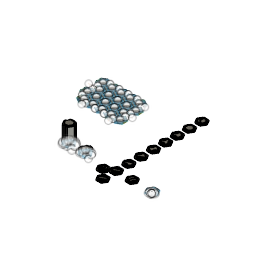
OpenHexTiles (Autodesk Fusion 360 design; units mm, degrees)
part number: 2025-10-27-16-40-17-945
part number: 2025-10-29-18-29-54-015
part number: 2025-10-29-18-44-09-003
part number: 2025-11-06-19-48-26-716
part number: 2025-11-07-19-21-59-291
part number: 2025-11-23-17-37-19-176
part number: 2025-11-23-17-48-45-361
part number: 2025-11-23-18-24-08-497
part number: 2025-11-24-19-12-39-372
part number: 2025-11-24-19-25-12-724
part number: 2025-11-24-19-31-14-734
part number: 2025-11-24-19-34-23-874
part number: 2025-11-24-19-39-51-757
part number: 2025-11-24-19-43-10-627
part number: 2025-11-24-19-46-33-060
part number: 2025-11-24-19-51-15-923
Autodesk Fusion 360 part; units mm, degrees
(part 1 of 3)
sketch "Main Hex Tile" plane through (0, 0, 0) normal (0, 0, 1) x (1, 0, 0) in component "Basic Hext Tile"
  line L0 (19.8352, 0.961) -> (10.3609, 17.371)
  line L1 (10.3609, 17.371) -> (-8.5878, 17.371)
  line L2 (-8.5878, 17.371) -> (-18.0621, 0.961)
  line L3 (-18.0621, 0.961) -> (-8.5878, -15.449)
  line L4 (-8.5878, -15.449) -> (10.3609, -15.449)
  line L5 (10.3609, -15.449) -> (19.8352, 0.961)
  line L6 (14.743, 0.961) -> (7.8148, 12.961)
  line L7 (7.8148, 12.961) -> (-6.0416, 12.961)
  line L8 (-6.0416, 12.961) -> (-12.9698, 0.961)
  line L9 (-12.9698, 0.961) -> (-6.0416, -11.039)
  line L10 (-6.0416, -11.039) -> (7.8148, -11.039)
  line L11 (7.8148, -11.039) -> (14.743, 0.961)
  line L12 (15.098, -7.244) -> (23.6888, -12.2039) construction
  line L13 (16.7724, -4.344) -> (13.4237, -10.144)
  line L14 (13.4237, -10.144) -> (14.9248, -12.744)
  line L15 (14.9248, -12.744) -> (19.7746, -4.344)
  line L16 (19.7746, -4.344) -> (16.7724, -4.344)
  line L17 (0.8866, -15.449) -> (0.8866, -15.2915) construction
  line L18 (0.8866, -15.2915) -> (0.8866, -9) construction
  line L19 (4.3866, -15.449) -> (6.1186, -12.449)
  line L20 (6.1186, -12.449) -> (-4.3455, -12.449)
  line L21 (-4.3455, -12.449) -> (-2.6134, -15.449)
  line L22 (5.7363, 19.971) -> (-3.9632, 19.971)
  line L23 (-3.9632, 19.971) -> (-2.4621, 17.371)
  line L24 (4.2352, 17.371) -> (5.7363, 19.971)
  line L25 (13.348, 12.1971) -> (9.8839, 12.1971)
  line L26 (9.8839, 12.1971) -> (15.116, 3.1349)
  line L27 (15.116, 3.1349) -> (16.848, 6.1349)
  line L28 (-18.0015, -4.344) -> (-13.1517, -12.744)
  line L29 (-13.1517, -12.744) -> (-11.6506, -10.144)
  line L30 (-14.9992, -4.344) -> (-18.0015, -4.344)
  line L31 (-15.0749, 6.1349) -> (-13.3429, 3.1349)
  line L32 (-13.3429, 3.1349) -> (-8.1108, 12.1971)
  line L33 (-8.1108, 12.1971) -> (-11.5749, 12.1971)
  line L34 (7.8725, 13.061) -> (-6.0994, 13.061)
  line L35 (-6.0994, 13.061) -> (-13.0853, 0.961)
  line L36 (-13.0853, 0.961) -> (-6.0994, -11.139)
  line L37 (-6.0994, -11.139) -> (7.8725, -11.139)
  line L38 (7.8725, -11.139) -> (14.8584, 0.961)
  line L39 (14.8584, 0.961) -> (7.8725, 13.061)
  point P0 (0.8866, 0.961)
  dimension "d4" = 32.82
  dimension "d29" = 5.8
  dimension "d31" = 2.6
  dimension "d32" = 60
  dimension "d34" = 7
  dimension "d35" = 60
  dimension "d37" = 360
  dimension "d44" = 3
  dimension "d59" = 0.1
  constraint horizontal L1
  constraint midpoint L5 L12.start
  constraint perpendicular L5 L12
  constraint perpendicular L12 L13
  constraint perpendicular L12 L15
  constraint midpoint L5 L13
  constraint symmetric L12 L14 L16
  constraint midpoint L4 L17.start
  constraint perpendicular L10 L17
  constraint perpendicular L10 L18
  constraint coincident L4 L21.end
  constraint coincident L4 L19.start
  constraint symmetric L18 L19 L21
  measures "d4" distance of L1 L4
  measures "d29" vertical distance of L13.start L13.end
  measures "d31" distance of L5 L15.end
  measures "d32" angle of L15 L16
  measures "d34" distance of L21.end L19.start
  measures "d35" angle of L20 L21
  measures "d44" distance of L4 L20
extrude "Dar Volumen" add sketch "Main Hex Tile" along normal blind 15 contours L0 L1 L2 L3 L4 L5 L13 L19 L20 L21 L25 L26 L27 L31 L32 L33 | L5 L13 L14 L15 L16 | L1 L22 L23 L24 | L3 L28 L29 L30 | L6 L7 L8 L9 L10 L11 | L34 L35 L36 L37 L38 L39 makes body 1 in component "Basic Hext Tile"
extrude "Recorte Labio Superior" cut sketch "Main Hex Tile" against normal blind 2 from surface at 15 contours L0 L1 L2 L3 L4 L5 L13 L19 L20 L21 L25 L26 L27 L31 L32 L33 | L5 L13 L14 L15 L16 | L1 L22 L23 L24 | L3 L28 L29 L30 | L34 L35 L36 L37 L38 L39 bodies 1 in component "Basic Hext Tile"
extrude "Machos" cut sketch "Main Hex Tile" along normal blind 6 contours L5 L13 L14 L15 L16 | L1 L22 L23 L24 | L3 L28 L29 L30 bodies 1 in component "Basic Hext Tile"
extrude "Extrude8" cut sketch "Main Hex Tile" along normal blind 11 contours L34 L35 L36 L37 L38 L39 bodies 1 in component "Basic Hext Tile"
extrude "Extrude9" cut sketch "Main Hex Tile" along normal blind 11 contours L6 L7 L8 L9 L10 L11 bodies 1 in component "Basic Hext Tile"
sketch "Basic Cap (Text)" plane through (0, 0, 0) normal (0, 0, 1) x (1, 0, 0) in component "Basic Cap (Text)"
  line L0 (30.6963, -0.205) -> (40.1706, -16.615)
  line L1 (40.1706, -16.615) -> (59.1192, -16.615)
  line L2 (59.1192, -16.615) -> (68.5936, -0.205)
  line L3 (68.5936, -0.205) -> (59.1192, 16.205)
  line L4 (59.1192, 16.205) -> (40.1706, 16.205)
  line L5 (40.1706, 16.205) -> (30.6963, -0.205)
  line L6 (42.7167, 11.795) -> (35.7885, -0.205)
  line L7 (35.7885, -0.205) -> (42.7167, -12.205)
  line L8 (42.7167, -12.205) -> (56.5731, -12.205)
  line L9 (56.5731, -12.205) -> (63.5013, -0.205)
  line L10 (63.5013, -0.205) -> (56.5731, 11.795)
  line L11 (56.5731, 11.795) -> (42.7167, 11.795)
  line L12 (42.659, 11.895) -> (35.6731, -0.205)
  line L13 (35.6731, -0.205) -> (42.659, -12.305)
  line L14 (42.659, -12.305) -> (56.6309, -12.305)
  line L15 (56.6309, -12.305) -> (63.6168, -0.205)
  line L16 (63.6168, -0.205) -> (56.6309, 11.895)
  line L17 (56.6309, 11.895) -> (42.659, 11.895)
  line L18 (36.7542, -3.3815) -> (62.5357, -3.3815) construction
  line L19 (62.5357, -3.3815) -> (62.5357, 2.9715) construction
  line L20 (62.5357, 2.9715) -> (36.7542, 2.9715) construction
  line L21 (36.7542, 2.9715) -> (36.7542, -3.3815) construction
  line L22 (49.6449, 11.795) -> (49.6449, -12.205) construction
  line L23 (60.0372, 5.795) -> (39.2526, -6.205) construction
  line L24 (39.166, 5.845) -> (60.1238, -6.255) construction
  line L25 (36.8278, -0.205) -> (43.2363, -11.305)
  line L26 (43.2363, -11.305) -> (56.0535, -11.305)
  line L27 (56.0535, -11.305) -> (62.4621, -0.205)
  line L28 (62.4621, -0.205) -> (56.0535, 10.895)
  line L29 (56.0535, 10.895) -> (43.2363, 10.895)
  line L30 (43.2363, 10.895) -> (36.8278, -0.205)
  point P0 (49.6449, -0.205)
  dimension "d65_1" = 32.82
  dimension "d67_1" = 0.1
  dimension "d88" = 4
  dimension "d89" = 0
  text T0 "+3\nWATER3\nPSR+1" font "Arial" height 4 bold align centre middle in box 25.7815 x 6.353 at (36.7542, -3.3815) x (1, 0) y (0, 1) spacing 1 kerned
  constraint horizontal L4
  constraint midpoint L11 L22.start
  constraint midpoint L8 L22.end
  constraint midpoint L10 L23.start
  constraint midpoint L7 L23.end
  constraint midpoint L12 L24.start
  constraint midpoint L15 L24.end
  constraint coincident P0
  constraint horizontal L20
  measures "d65_1" distance of L1 L4
extrude "Main Cap Body" add sketch "Basic Cap (Text)" sketch "Basic Cap (Text)" along normal blind 4.8 separate body contours L0 L1 L2 L3 L4 L5 | L6 L7 L8 L9 L10 L11 | L12 L13 L14 L15 L16 L17 | L25 L26 L27 L28 L29 L30 of sketch 2 text T0 makes body 2 in component "Basic Cap (Text)"
extrude "Outside lip cut" cut sketch "Basic Cap (Text)" against normal blind 1.8 from surface at 4.8 contours L0 L1 L2 L3 L4 L5 | L12 L13 L14 L15 L16 L17 bodies 2 in component "Basic Cap (Text)"
extrude "Hole for text" cut sketch "Basic Cap (Text)" against normal blind 1.2 from surface at 4.8 contours L25 L26 L27 L28 L29 L30 bodies 2 in component "Basic Cap (Text)"
extrude "Internal Hole" cut sketch "Basic Cap (Text)" along normal blind 2 contours L6 L7 L8 L9 L10 L11 | L12 L13 L14 L15 L16 L17 | L25 L26 L27 L28 L29 L30 bodies 2 in component "Basic Cap (Text)"
extrude "Text" add sketch "Basic Cap (Text)" along normal blind 1.2 from surface at 3.6 text T0 bodies 2 in component "Basic Cap (Text)"
sketch "Slab" plane through (0, 0, 0) normal (0, 0, 1) x (1, 0, 0) in component "Slab"
  line L0 (-173.2109, 149.9603) -> (-156.8009, 159.4346)
  line L1 (-189.6209, 178.3833) -> (-189.6209, 159.4346)
  line L2 (-189.6209, 159.4346) -> (-173.2109, 149.9603)
  line L3 (-185.2109, 175.8372) -> (-185.2109, 161.9807)
  line L4 (-185.2109, 161.9807) -> (-173.2109, 155.0525)
  line L5 (-173.2109, 155.0525) -> (-161.2109, 161.9807)
  line L6 (-161.2109, 161.9807) -> (-161.2109, 175.8372)
  line L7 (-161.2109, 175.8372) -> (-173.2109, 182.7654)
  line L8 (-173.2109, 182.7654) -> (-185.2109, 175.8372)
  line L9 (-152.3909, 175.8372) -> (-152.3909, 161.9807)
  line L10 (-140.3909, 182.7654) -> (-152.3909, 175.8372)
  line L11 (-128.3909, 175.8372) -> (-140.3909, 182.7654)
  line L12 (-152.3909, 161.9807) -> (-140.3909, 155.0525)
  line L13 (-140.3909, 155.0525) -> (-128.3909, 161.9807)
  line L14 (-128.3909, 161.9807) -> (-128.3909, 175.8372)
  line L15 (-156.8009, 159.4346) -> (-140.3909, 149.9603)
  line L16 (-140.3909, 149.9603) -> (-123.9809, 159.4346)
  line L17 (-119.5709, 175.8372) -> (-119.5709, 161.9807)
  line L18 (-107.5709, 182.7654) -> (-119.5709, 175.8372)
  line L19 (-95.5709, 175.8372) -> (-107.5709, 182.7654)
  line L20 (-119.5709, 161.9807) -> (-107.5709, 155.0525)
  line L21 (-107.5709, 155.0525) -> (-95.5709, 161.9807)
  line L22 (-95.5709, 161.9807) -> (-95.5709, 175.8372)
  line L23 (-123.9809, 159.4346) -> (-107.5709, 149.9603)
  line L24 (-107.5709, 149.9603) -> (-91.1609, 159.4346)
  line L25 (-86.7509, 175.8372) -> (-86.7509, 161.9807)
  line L26 (-74.7509, 182.7654) -> (-86.7509, 175.8372)
  line L27 (-62.7509, 175.8372) -> (-74.7509, 182.7654)
  line L28 (-86.7509, 161.9807) -> (-74.7509, 155.0525)
  line L29 (-74.7509, 155.0525) -> (-62.7509, 161.9807)
  line L30 (-62.7509, 161.9807) -> (-62.7509, 175.8372)
  line L31 (-91.1609, 159.4346) -> (-74.7509, 149.9603)
  line L32 (-74.7509, 149.9603) -> (-58.3409, 159.4346)
  line L33 (-53.9309, 175.8372) -> (-53.9309, 161.9807)
  line L34 (-41.9309, 182.7654) -> (-53.9309, 175.8372)
  line L35 (-29.9309, 175.8372) -> (-41.9309, 182.7654)
  line L36 (-25.5209, 178.3833) -> (-41.9309, 187.8576)
  line L37 (-53.9309, 161.9807) -> (-41.9309, 155.0525)
  line L38 (-41.9309, 155.0525) -> (-29.9309, 161.9807)
  line L39 (-29.9309, 161.9807) -> (-29.9309, 175.8372)
  line L40 (-58.3409, 159.4346) -> (-41.9309, 149.9603)
  line L41 (-25.5209, 159.4346) -> (-25.5209, 178.3833)
  line L42 (-41.9309, 149.9603) -> (-25.5209, 159.4346)
  line L43 (-189.6209, 216.2805) -> (-206.0309, 206.8062)
  line L44 (-206.0309, 206.8062) -> (-206.0309, 187.8576)
  line L45 (-206.0309, 187.8576) -> (-189.6209, 178.3833)
  line L46 (-201.6209, 204.2601) -> (-201.6209, 190.4037)
  line L47 (-201.6209, 190.4037) -> (-189.6209, 183.4755)
  line L48 (-189.6209, 183.4755) -> (-177.6209, 190.4037)
  line L49 (-177.6209, 190.4037) -> (-177.6209, 204.2601)
  line L50 (-177.6209, 204.2601) -> (-189.6209, 211.1883)
  line L51 (-189.6209, 211.1883) -> (-201.6209, 204.2601)
  line L52 (-144.8009, 204.2601) -> (-156.8009, 211.1883)
  line L53 (-168.8009, 204.2601) -> (-168.8009, 190.4037)
  line L54 (-144.8009, 190.4037) -> (-144.8009, 204.2601)
  line L55 (-156.8009, 183.4755) -> (-144.8009, 190.4037)
  line L56 (-168.8009, 190.4037) -> (-156.8009, 183.4755)
  line L57 (-156.8009, 211.1883) -> (-168.8009, 204.2601)
  line L58 (-111.9809, 204.2601) -> (-123.9809, 211.1883)
  line L59 (-135.9809, 204.2601) -> (-135.9809, 190.4037)
  line L60 (-111.9809, 190.4037) -> (-111.9809, 204.2601)
  line L61 (-123.9809, 183.4755) -> (-111.9809, 190.4037)
  line L62 (-135.9809, 190.4037) -> (-123.9809, 183.4755)
  line L63 (-123.9809, 211.1883) -> (-135.9809, 204.2601)
  line L64 (-79.1609, 204.2601) -> (-91.1609, 211.1883)
  line L65 (-103.1609, 204.2601) -> (-103.1609, 190.4037)
  line L66 (-79.1609, 190.4037) -> (-79.1609, 204.2601)
  line L67 (-91.1609, 183.4755) -> (-79.1609, 190.4037)
  line L68 (-103.1609, 190.4037) -> (-91.1609, 183.4755)
  line L69 (-91.1609, 211.1883) -> (-103.1609, 204.2601)
  line L70 (-46.3409, 204.2601) -> (-58.3409, 211.1883)
  line L71 (-70.3409, 204.2601) -> (-70.3409, 190.4037)
  line L72 (-46.3409, 190.4037) -> (-46.3409, 204.2601)
  line L73 (-41.9309, 187.8576) -> (-41.9309, 206.8062)
  line L74 (-58.3409, 183.4755) -> (-46.3409, 190.4037)
  line L75 (-70.3409, 190.4037) -> (-58.3409, 183.4755)
  line L76 (-58.3409, 211.1883) -> (-70.3409, 204.2601)
  line L77 (-128.3909, 218.8266) -> (-128.3909, 232.683)
  line L78 (-201.6209, 261.106) -> (-201.6209, 247.2496)
  line L79 (-140.3909, 211.8984) -> (-128.3909, 218.8266)
  line L80 (-168.8009, 261.106) -> (-168.8009, 247.2496)
  line L81 (-86.7509, 218.8266) -> (-74.7509, 211.8984)
  line L82 (-152.3909, 218.8266) -> (-140.3909, 211.8984)
  line L83 (-95.5709, 218.8266) -> (-95.5709, 232.683)
  line L84 (-189.6209, 235.2292) -> (-189.6209, 216.2805)
  line L85 (-206.0309, 263.6521) -> (-206.0309, 244.7035)
  line L86 (-177.6209, 247.2496) -> (-177.6209, 261.106)
  line L87 (-189.6209, 268.0342) -> (-201.6209, 261.106)
  line L88 (-156.8009, 273.1264) -> (-173.2109, 263.6521)
  line L89 (-201.6209, 247.2496) -> (-189.6209, 240.3214)
  line L90 (-144.8009, 247.2496) -> (-144.8009, 261.106)
  line L91 (-173.2109, 263.6521) -> (-189.6209, 273.1264)
  line L92 (-74.7509, 211.8984) -> (-62.7509, 218.8266)
  line L93 (-119.5709, 232.683) -> (-119.5709, 218.8266)
  line L94 (-86.7509, 232.683) -> (-86.7509, 218.8266)
  line L95 (-156.8009, 240.3214) -> (-144.8009, 247.2496)
  line L96 (-140.3909, 263.6521) -> (-156.8009, 273.1264)
  line L97 (-62.7509, 218.8266) -> (-62.7509, 232.683)
  line L98 (-107.5709, 211.8984) -> (-95.5709, 218.8266)
  line L99 (-168.8009, 247.2496) -> (-156.8009, 240.3214)
  line L100 (-152.3909, 232.683) -> (-152.3909, 218.8266)
  line L101 (-185.2109, 232.683) -> (-185.2109, 218.8266)
  line L102 (-111.9809, 247.2496) -> (-111.9809, 261.106)
  line L103 (-173.2109, 211.8984) -> (-161.2109, 218.8266)
  line L104 (-185.2109, 218.8266) -> (-173.2109, 211.8984)
  line L105 (-135.9809, 247.2496) -> (-123.9809, 240.3214)
  line L106 (-161.2109, 218.8266) -> (-161.2109, 232.683)
  line L107 (-123.9809, 273.1264) -> (-140.3909, 263.6521)
  line L108 (-119.5709, 218.8266) -> (-107.5709, 211.8984)
  line L109 (-111.9809, 261.106) -> (-123.9809, 268.0342)
  line L110 (-107.5709, 263.6521) -> (-123.9809, 273.1264)
  line L111 (-177.6209, 261.106) -> (-189.6209, 268.0342)
  line L112 (-79.1609, 247.2496) -> (-79.1609, 261.106)
  line L113 (-144.8009, 261.106) -> (-156.8009, 268.0342)
  line L114 (-156.8009, 268.0342) -> (-168.8009, 261.106)
  line L115 (-189.6209, 273.1264) -> (-206.0309, 263.6521)
  line L116 (-103.1609, 261.106) -> (-103.1609, 247.2496)
  line L117 (-123.9809, 240.3214) -> (-111.9809, 247.2496)
  line L118 (-189.6209, 240.3214) -> (-177.6209, 247.2496)
  line L119 (-123.9809, 268.0342) -> (-135.9809, 261.106)
  line L120 (-135.9809, 261.106) -> (-135.9809, 247.2496)
  line L121 (-91.1609, 273.1264) -> (-107.5709, 263.6521)
  line L122 (-46.3409, 261.106) -> (-58.3409, 268.0342)
  line L123 (-25.5209, 235.2292) -> (-41.9309, 244.7035)
  line L124 (-29.9309, 232.683) -> (-41.9309, 239.6112)
  line L125 (-107.5709, 239.6112) -> (-119.5709, 232.683)
  line L126 (-58.3409, 240.3214) -> (-46.3409, 247.2496)
  line L127 (-41.9309, 239.6112) -> (-53.9309, 232.683)
  line L128 (-74.7509, 239.6112) -> (-86.7509, 232.683)
  line L129 (-103.1609, 247.2496) -> (-91.1609, 240.3214)
  line L130 (-41.9309, 263.6521) -> (-58.3409, 273.1264)
  line L131 (-70.3409, 261.106) -> (-70.3409, 247.2496)
  line L132 (-74.7509, 263.6521) -> (-91.1609, 273.1264)
  line L133 (-29.9309, 218.8266) -> (-29.9309, 232.683)
  line L134 (-46.3409, 247.2496) -> (-46.3409, 261.106)
  line L135 (-41.9309, 244.7035) -> (-41.9309, 263.6521)
  line L136 (-53.9309, 232.683) -> (-53.9309, 218.8266)
  line L137 (-91.1609, 268.0342) -> (-103.1609, 261.106)
  line L138 (-41.9309, 211.8984) -> (-29.9309, 218.8266)
  line L139 (-128.3909, 232.683) -> (-140.3909, 239.6112)
  line L140 (-79.1609, 261.106) -> (-91.1609, 268.0342)
  line L141 (-25.5209, 216.2805) -> (-25.5209, 235.2292)
  line L142 (-173.2109, 239.6112) -> (-185.2109, 232.683)
  line L143 (-91.1609, 240.3214) -> (-79.1609, 247.2496)
  line L144 (-62.7509, 232.683) -> (-74.7509, 239.6112)
  line L145 (-140.3909, 239.6112) -> (-152.3909, 232.683)
  line L146 (-53.9309, 218.8266) -> (-41.9309, 211.8984)
  line L147 (-41.9309, 206.8062) -> (-25.5209, 216.2805)
  line L148 (-206.0309, 244.7035) -> (-189.6209, 235.2291)
  line L149 (-95.5709, 232.683) -> (-107.5709, 239.6112)
  line L150 (-161.2109, 232.683) -> (-173.2109, 239.6112)
  line L151 (-58.3409, 273.1264) -> (-74.7509, 263.6521)
  line L152 (-70.3409, 247.2496) -> (-58.3409, 240.3214)
  line L153 (-58.3409, 268.0342) -> (-70.3409, 261.106)
  line L154 (-41.9309, 254.1778) -> (-36.7309, 254.1778) construction
  line L155 (-41.9309, 197.3319) -> (-25.9796, 197.3319) construction
  line L156 (-25.5209, 225.7548) -> (-29.9309, 225.7548) construction
  line L157 (-25.5209, 168.909) -> (-29.9309, 168.909) construction
  line L158 (-206.0309, 254.1778) -> (-201.6209, 254.1778) construction
  line L159 (-206.0309, 197.3319) -> (-201.6209, 197.3319) construction
  line L160 (-189.6209, 225.7548) -> (-213.2603, 225.7548) construction
  line L161 (-165.0059, 154.6975) -> (-161.3598, 148.3824) construction
  line L162 (-66.5459, 154.6975) -> (-60.8001, 144.7456) construction
  line L163 (-66.5459, 268.3893) -> (-64.3409, 264.5701) construction
  line L164 (-165.0059, 268.3893) -> (-162.8009, 264.5701) construction
  line L165 (-41.9309, 200.2319) -> (-39.3309, 201.733)
  line L166 (-39.3309, 201.733) -> (-39.3309, 192.9308)
  line L167 (-39.3309, 192.9308) -> (-41.9309, 194.4319)
  line L168 (-41.9309, 257.0778) -> (-39.3309, 258.5789)
  line L169 (-39.3309, 258.5789) -> (-39.3309, 249.7767)
  line L170 (-39.3309, 249.7767) -> (-41.9309, 251.2778)
  line L171 (-64.0344, 156.1475) -> (-61.4344, 154.6464)
  line L172 (-61.4344, 154.6464) -> (-69.0573, 150.2453)
  line L173 (-69.0573, 150.2453) -> (-69.0573, 153.2475)
  line L174 (-162.4944, 156.1475) -> (-159.8944, 154.6464)
  line L175 (-159.8944, 154.6464) -> (-167.5173, 150.2453)
  line L176 (-167.5173, 150.2453) -> (-167.5173, 153.2475)
  line L177 (-206.0309, 200.8319) -> (-203.2309, 202.4485)
  line L178 (-203.2309, 202.4485) -> (-203.2309, 192.2153)
  line L179 (-203.2309, 192.2153) -> (-206.0309, 193.8319)
  line L180 (-206.0309, 257.6778) -> (-203.2309, 259.2944)
  line L181 (-203.2309, 259.2944) -> (-203.2309, 249.0612)
  line L182 (-203.2309, 249.0612) -> (-206.0309, 250.6778)
  line L183 (-168.037, 266.6393) -> (-168.037, 263.4061)
  line L184 (-168.037, 263.4061) -> (-159.1748, 268.5227)
  line L185 (-159.1748, 268.5227) -> (-161.9748, 270.1393)
  line L186 (-69.577, 266.6393) -> (-69.577, 263.4061)
  line L187 (-69.577, 263.4061) -> (-60.7148, 268.5227)
  line L188 (-60.7148, 268.5227) -> (-63.5148, 270.1393)
  point P0 (-173.2109, 168.909)
  point P1 (-140.3909, 168.909)
  point P2 (-107.5709, 168.909)
  point P3 (-74.7509, 168.909)
  point P4 (-41.9309, 168.909)
  point P5 (-189.6209, 197.3319)
  point P6 (-156.8009, 197.3319)
  point P7 (-123.9809, 197.3319)
  point P8 (-91.1609, 197.3319)
  point P9 (-58.3409, 197.3319)
  point P10 (-74.7509, 225.7548)
  point P11 (-173.2109, 225.7548)
  point P12 (-41.9309, 225.7548)
  point P13 (-156.8009, 254.1778)
  point P14 (-123.9809, 254.1778)
  point P15 (-107.5709, 225.7548)
  point P16 (-140.3909, 225.7548)
  point P17 (-91.1609, 254.1778)
  point P18 (-189.6209, 254.1778)
  point P19 (-58.3409, 254.1778)
  dimension "d257" = 16.41
  dimension "d258" = 28.4229
  dimension "d268" = 2.6
  dimension "d269" = 60
  dimension "d270" = 5.8
  dimension "d274" = 60
  dimension "d275" = 5.8
  dimension "d276" = 2.6
  dimension "d277" = 60
  dimension "d278" = 2.6
  dimension "d279" = 5.8
  dimension "d280" = 60
  dimension "d281" = 5.8
  dimension "d282" = 2.6
  dimension "d295" = 7
  dimension "d296" = 2.8
  dimension "d297" = 60
  dimension "d298" = 7
  dimension "d299" = 2.8
  dimension "d300" = 60
  dimension "d301" = 7
  dimension "d302" = 2.8
  dimension "d303" = 60
  dimension "d304" = 7
  dimension "d305" = 2.8
  dimension "d306" = 60
  constraint midpoint L135 L154.start
  constraint perpendicular L135 L154
  constraint midpoint L73 L155.start
  constraint perpendicular L73 L155
  constraint midpoint L141 L156.start
  constraint midpoint L133 L156.end
  constraint midpoint L41 L157.start
  constraint midpoint L39 L157.end
  constraint midpoint L85 L158.start
  constraint midpoint L78 L158.end
  constraint midpoint L44 L159.start
  constraint midpoint L46 L159.end
  constraint midpoint L84 L160.start
  constraint perpendicular L84 L160
  constraint midpoint L0 L161.start
  constraint perpendicular L0 L161
  constraint midpoint L32 L162.start
  constraint perpendicular L32 L162
  constraint midpoint L151 L163.start
  constraint midpoint L153 L163.end
  constraint midpoint L88 L164.start
  constraint midpoint L114 L164.end
  constraint coincident L73 L165.start
  constraint perpendicular L155 L166
  constraint coincident L73 L167.end
  constraint symmetric L155 L165 L167
  constraint coincident L135 L168.start
  constraint perpendicular L154 L169
  constraint coincident L135 L170.end
  constraint symmetric L154 L168 L170
  constraint coincident L32 L171.start
  constraint perpendicular L162 L172
  constraint coincident L32 L173.end
  constraint symmetric L162 L171 L173
  constraint coincident L0 L174.start
  constraint coincident L0 L176.end
  constraint vertical L176
  constraint parallel L0 L175
  constraint symmetric L161 L174 L176
  constraint coincident L44 L177.start
  constraint perpendicular L159 L178
  constraint coincident L44 L179.end
  constraint symmetric L159 L177 L179
  constraint coincident L85 L180.start
  constraint perpendicular L158 L181
  constraint coincident L85 L182.end
  constraint symmetric L158 L180 L182
  constraint coincident L88 L183.start
  constraint perpendicular L164 L184
  constraint coincident L88 L185.end
  constraint symmetric L164 L183 L185
  constraint coincident L151 L186.start
  constraint perpendicular L163 L187
  constraint coincident L151 L188.end
  constraint symmetric L163 L186 L188
  measures "d257" horizontal distance of P0 P5
  measures "d258" vertical distance of P0 P5
  measures "d268" distance of L73 L166
  measures "d269" angle of L73 L165
  measures "d270" distance of L165.start L167.end
  measures "d274" angle of L135 L168
  measures "d275" distance of L168.start L170.end
  measures "d276" distance of L135 L169
  measures "d277" angle of L32 L171
  measures "d278" distance of L32 L172
  measures "d279" distance of L171.start L173.end
  measures "d280" angle of L0 L174
  measures "d281" distance of L174.start L176.end
  measures "d282" distance of L0 L175
  measures "d295" distance of L177.start L179.end
  measures "d296" distance of L44 L178
  measures "d297" angle of L44 L177
  measures "d298" distance of L180.start L182.end
  measures "d299" distance of L85 L181
  measures "d300" angle of L85 L180
  measures "d301" distance of L183.start L185.end
  measures "d302" distance of L88 L184
  measures "d303" angle of L88 L185
  measures "d304" distance of L186.start L188.end
  measures "d305" distance of L151 L187
  measures "d306" angle of L151 L188
extrude "slab body" add sketch "Slab" along normal blind 2 separate body contours L0 L1 L2 L15 L16 L23 L24 L31 L32 L36 L40 L41 L42 L43 L44 L45 L73 L84 L85 L88 L91 L96 L107 L110 L115 L121 L123 L130 L132 L135 L141 L147 L148 L151 L177 L178 L179 L180 L181 L182 L183 L184 L185 L186 L187 L188 | L0 L174 L175 L176 | L32 L171 L172 L173 | L73 L165 L166 L167 | L135 L168 L169 L170 | L3 L4 L5 L6 L7 L8 | L9 L10 L11 L12 L13 L14 | L17 L18 L19 L20 L21 L22 | L25 L26 L27 L28 L29 L30 | L33 L34 L35 L37 L38 L39 | L46 L47 L48 L49 L50 L51 | L52 L53 L54 L55 L56 L57 | L58 L59 L60 L61 L62 L63 | L64 L65 L66 L67 L68 L69 | L70 L71 L72 L74 L75 L76 | L77 L79 L82 L100 L139 L145 | L78 L86 L87 L89 L111 L118 | L80 L90 L95 L99 L113 L114 | L81 L92 L94 L97 L128 L144 | L83 L93 L98 L108 L125 L149 | L101 L103 L104 L106 L142 L150 | L102 L105 L109 L117 L119 L120 | L112 L116 L129 L137 L140 L143 | L122 L126 L131 L134 L152 L153 | L124 L127 L133 L136 L138 L146 makes body 3 in component "Slab"
extrude "slab tops" add sketch "Slab" along normal blind 2 from surface at 2 contours L3 L4 L5 L6 L7 L8 | L9 L10 L11 L12 L13 L14 | L17 L18 L19 L20 L21 L22 | L25 L26 L27 L28 L29 L30 | L33 L34 L35 L37 L38 L39 | L46 L47 L48 L49 L50 L51 | L52 L53 L54 L55 L56 L57 | L58 L59 L60 L61 L62 L63 | L64 L65 L66 L67 L68 L69 | L70 L71 L72 L74 L75 L76 | L77 L79 L82 L100 L139 L145 | L78 L86 L87 L89 L111 L118 | L80 L90 L95 L99 L113 L114 | L81 L92 L94 L97 L128 L144 | L83 L93 L98 L108 L125 L149 | L101 L103 L104 L106 L142 L150 | L102 L105 L109 L117 L119 L120 | L112 L116 L129 L137 L140 L143 | L122 L126 L131 L134 L152 L153 | L124 L127 L133 L136 L138 L146 bodies 3 in component "Slab"
sketch "Multi Height Hex" plane through (0, 0, 0) normal (0, 0, 1) x (1, 0, 0) in component "Multi height Hex"
  line L0 (19.8352, 0.961) -> (10.3609, 17.371)
  line L1 (10.3609, 17.371) -> (-8.5878, 17.371)
  line L2 (-8.5878, 17.371) -> (-18.0621, 0.961)
  line L3 (-18.0621, 0.961) -> (-8.5878, -15.449)
  line L4 (-8.5878, -15.449) -> (10.3609, -15.449)
  line L5 (10.3609, -15.449) -> (19.8352, 0.961)
  line L6 (14.743, 0.961) -> (7.8148, 12.961)
  line L7 (7.8148, 12.961) -> (-6.0416, 12.961)
  line L8 (-6.0416, 12.961) -> (-12.9698, 0.961)
  line L9 (-12.9698, 0.961) -> (-6.0416, -11.039)
  line L10 (-6.0416, -11.039) -> (7.8148, -11.039)
  line L11 (7.8148, -11.039) -> (14.743, 0.961)
  line L12 (15.098, -7.244) -> (23.6888, -12.2039) construction
  line L13 (16.7724, -4.344) -> (13.4237, -10.144)
  line L14 (13.4237, -10.144) -> (14.9248, -12.744)
  line L15 (14.9248, -12.744) -> (19.7746, -4.344)
  line L16 (19.7746, -4.344) -> (16.7724, -4.344)
  line L17 (0.8866, -15.449) -> (0.8866, -15.2915) construction
  line L18 (0.8866, -15.2915) -> (0.8866, -9) construction
  line L19 (4.3866, -15.449) -> (6.1186, -12.449)
  line L20 (6.1186, -12.449) -> (-4.3455, -12.449)
  line L21 (-4.3455, -12.449) -> (-2.6134, -15.449)
  line L22 (5.7363, 19.971) -> (-3.9632, 19.971)
  line L23 (-3.9632, 19.971) -> (-2.4621, 17.371)
  line L24 (4.2352, 17.371) -> (5.7363, 19.971)
  line L25 (13.348, 12.1971) -> (9.8839, 12.1971)
  line L26 (9.8839, 12.1971) -> (15.116, 3.1349)
  line L27 (15.116, 3.1349) -> (16.848, 6.1349)
  line L28 (-18.0015, -4.344) -> (-13.1517, -12.744)
  line L29 (-13.1517, -12.744) -> (-11.6506, -10.144)
  line L30 (-14.9992, -4.344) -> (-18.0015, -4.344)
  line L31 (-15.0749, 6.1349) -> (-13.3429, 3.1349)
  line L32 (-13.3429, 3.1349) -> (-8.1108, 12.1971)
  line L33 (-8.1108, 12.1971) -> (-11.5749, 12.1971)
  line L34 (7.8725, 13.061) -> (-6.0994, 13.061)
  line L35 (-6.0994, 13.061) -> (-13.0853, 0.961)
  line L36 (-13.0853, 0.961) -> (-6.0994, -11.139)
  line L37 (-6.0994, -11.139) -> (7.8725, -11.139)
  line L38 (7.8725, -11.139) -> (14.8584, 0.961)
  line L39 (14.8584, 0.961) -> (7.8725, 13.061)
  point P0 (0.8866, 0.961)
  dimension "d4_1" = 32.82
  dimension "d29_1" = 5.8
  dimension "d31_1" = 2.6
  dimension "d32_1" = 60
  dimension "d34_1" = 7
  dimension "d35_1" = 60
  dimension "d37_1" = 360
  dimension "d44_1" = 3
  dimension "d59_1" = 0.1
  constraint horizontal L1
  constraint midpoint L5 L12.start
  constraint perpendicular L5 L12
  constraint perpendicular L12 L13
  constraint perpendicular L12 L15
  constraint midpoint L5 L13
  constraint symmetric L12 L14 L16
  constraint midpoint L4 L17.start
  constraint perpendicular L10 L17
  constraint perpendicular L10 L18
  constraint coincident L4 L21.end
  constraint coincident L4 L19.start
  constraint symmetric L18 L19 L21
  measures "d4_1" distance of L1 L4
  measures "d29_1" vertical distance of L13.start L13.end
  measures "d31_1" distance of L5 L15.end
  measures "d32_1" angle of L15 L16
  measures "d34_1" distance of L21.end L19.start
  measures "d35_1" angle of L20 L21
  measures "d44_1" distance of L4 L20
extrude "Dar Volumen'" add sketch "Multi Height Hex" along normal blind 67 separate body contours L0 L1 L2 L3 L4 L5 L13 L19 L20 L21 L25 L26 L27 L31 L32 L33 | L5 L13 L14 L15 L16 | L1 L22 L23 L24 | L3 L28 L29 L30 | L6 L7 L8 L9 L10 L11 | L34 L35 L36 L37 L38 L39 makes body 4 in component "Multi height Hex"
extrude "Bottom Male DoveTail Cut" cut sketch "Multi Height Hex" along normal blind 6 contours L5 L13 L14 L15 L16 | L1 L22 L23 L24 | L3 L28 L29 L30 bodies 4 in component "Multi height Hex"
extrude "Top Male Dovetail Cut" cut sketch "Multi Height Hex" against normal blind 54 from surface at 67 contours L5 L13 L14 L15 L16 | L1 L22 L23 L24 | L3 L28 L29 L30 bodies 4 in component "Multi height Hex"
extrude "Top Lip Cut" cut sketch "Multi Height Hex" against normal blind 2 from surface at 67 contours L0 L1 L2 L3 L4 L5 L13 L19 L20 L21 L25 L26 L27 L31 L32 L33 | L34 L35 L36 L37 L38 L39 bodies 4 in component "Multi height Hex"
extrude "Internal Hole'" cut sketch "Multi Height Hex" along normal blind 63 contours L6 L7 L8 L9 L10 L11 | L34 L35 L36 L37 L38 L39 bodies 4 in component "Multi height Hex"
sketch "Road Cap" plane through (0, 0, 0) normal (0, 0, 1) x (1, 0, 0) in component "Road Cap"
  line L0 (106.7167, 11.795) -> (99.7885, -0.205)
  line L1 (120.6309, 11.895) -> (106.659, 11.895)
  line L2 (106.7167, -12.205) -> (120.5731, -12.205)
  line L3 (104.1706, -16.615) -> (123.1192, -16.615)
  line L4 (120.0535, -11.305) -> (126.4621, -0.205)
  line L5 (99.6731, -0.205) -> (106.659, -12.305)
  line L6 (94.6963, -0.205) -> (104.1706, -16.615)
  line L7 (100.8278, -0.205) -> (107.2363, -11.305)
  line L8 (107.2363, -11.305) -> (120.0535, -11.305)
  line L9 (132.5936, -0.205) -> (123.1192, 16.205)
  line L10 (127.5013, -0.205) -> (120.5731, 11.795)
  line L11 (124.0372, 5.795) -> (103.2526, -6.205) construction
  line L12 (104.1706, 16.205) -> (94.6963, -0.205)
  line L13 (103.166, 5.845) -> (124.1238, -6.255) construction
  line L14 (106.659, -12.305) -> (120.6309, -12.305)
  line L15 (120.6309, -12.305) -> (127.6168, -0.205)
  line L16 (120.5731, 11.795) -> (106.7167, 11.795)
  line L17 (127.6168, -0.205) -> (120.6309, 11.895)
  line L18 (123.1192, -16.615) -> (132.5936, -0.205)
  line L19 (123.1192, 16.205) -> (104.1706, 16.205)
  line L20 (126.4621, -0.205) -> (120.0535, 10.895)
  line L21 (120.5731, -12.205) -> (127.5013, -0.205)
  line L22 (106.659, 11.895) -> (99.6731, -0.205)
  line L23 (120.0535, 10.895) -> (107.2363, 10.895)
  line L24 (113.6449, 11.795) -> (113.6449, -12.205) construction
  line L25 (107.2363, 10.895) -> (100.8278, -0.205)
  line L26 (99.7885, -0.205) -> (106.7167, -12.205)
  line L27 (101.532, -1.4249) -> (120.7578, 9.6751)
  line L28 (106.532, -10.0851) -> (125.7578, 1.0149)
  line L29 (101.732, -1.7713) -> (120.9578, 9.3287)
  line L30 (106.332, -9.7387) -> (125.5578, 1.3613)
  point P0 (113.6449, -0.205)
  dimension "d328" = 0.1
  dimension "d330" = 32.82
  dimension "d366" = 10
  dimension "d369" = 0.4
  constraint horizontal L19
  constraint midpoint L24.start L16
  constraint midpoint L24.end L2
  constraint midpoint L11.start L10
  constraint midpoint L11.end L26
  constraint midpoint L13.start L22
  constraint midpoint L13.end L15
  constraint coincident L7 L27.start
  constraint coincident L20 L27.end
  constraint perpendicular L20 L27
  constraint coincident L7 L28.start
  constraint coincident L20 L28.end
  constraint perpendicular L20 L28
  constraint symmetric L11 L27 L28
  measures "d330" distance of L3 L19
  measures "d366" distance of L27 L28
extrude "cap body" add sketch "Road Cap" along normal blind 4.8 separate body contours L0 L2 L10 L16 L21 L26 | L1 L5 L14 L15 L17 L22 | L3 L6 L9 L12 L18 L19 | L4 L7 L8 L20 L28 | L7 L20 L28 L30 | L7 L20 L29 L30 | L7 L20 L27 L29 | L7 L20 L23 L25 L27 makes body 5 in component "Road Cap"
extrude "top lip cut" cut sketch "Road Cap" against normal blind 1.8 from surface at 4.8 contours L1 L5 L14 L15 L17 L22 | L3 L6 L9 L12 L18 L19 bodies 5 in component "Road Cap"
sketch "Road Cap Curve" plane through (0, 0, 0) normal (0, 0, 1) x (1, 0, 0) in component "Road Cap Curve"
  line L0 (106.898, 12.0938) -> (99.9698, 0.0938)
  line L1 (120.8122, 12.1938) -> (106.8403, 12.1938)
  line L2 (106.898, -11.9062) -> (120.7544, -11.9062)
  line L3 (104.3519, -16.3162) -> (123.3006, -16.3162)
  line L4 (120.2348, -11.0062) -> (126.6434, 0.0938)
  line L5 (99.8544, 0.0938) -> (106.8403, -12.0062)
  line L6 (94.8776, 0.0938) -> (104.3519, -16.3162)
  line L7 (101.0091, 0.0938) -> (107.4176, -11.0062)
  line L8 (107.4176, -11.0062) -> (120.2348, -11.0062)
  line L9 (132.7749, 0.0938) -> (123.3006, 16.5038)
  line L10 (127.6826, 0.0938) -> (120.7544, 12.0938)
  line L11 (124.2185, 6.0938) -> (103.4339, -5.9062) construction
  line L12 (104.3519, 16.5038) -> (94.8776, 0.0938)
  line L13 (103.3473, 6.1438) -> (124.3051, -5.9562) construction
  line L14 (106.8403, -12.0062) -> (120.8122, -12.0062)
  line L15 (120.8122, -12.0062) -> (127.7981, 0.0938)
  line L16 (120.7544, 12.0938) -> (106.898, 12.0938)
  line L17 (127.7981, 0.0938) -> (120.8122, 12.1938)
  line L18 (123.3006, -16.3162) -> (132.7749, 0.0938)
  line L19 (123.3006, 16.5038) -> (104.3519, 16.5038)
  line L20 (126.6434, 0.0938) -> (120.2348, 11.1938)
  line L21 (120.7544, -11.9062) -> (127.6826, 0.0938)
  line L22 (106.8403, 12.1938) -> (99.8544, 0.0938)
  line L23 (120.2348, 11.1938) -> (107.4176, 11.1938)
  line L24 (113.8262, 12.0938) -> (113.8262, -11.9062) construction
  line L25 (107.4176, 11.1938) -> (101.0091, 0.0938)
  line L26 (99.9698, 0.0938) -> (106.898, -11.9062)
  arc A0 (124.2185, 6.0938) -> (113.8262, -11.9062) centre (134.6108, -11.9062) ccw
  arc A1 (121.7185, 10.4239) -> (108.8262, -11.9062) centre (134.6108, -11.9062) ccw
  arc A2 (126.7185, 1.7637) -> (118.8262, -11.9062) centre (134.6108, -11.9062) ccw
  arc A3 (121.9185, 10.0775) -> (109.2262, -11.9062) centre (134.6108, -11.9062) ccw
  arc A4 (126.5185, 2.1101) -> (118.4262, -11.9062) centre (134.6108, -11.9062) ccw
  point P0 (113.8262, 0.0938)
  dimension "d328_1" = 0.1
  dimension "d330_1" = 32.82
  dimension "d395" = 5
  dimension "d396" = -5
  dimension "d398" = 0.4
  constraint horizontal L19
  constraint midpoint L24.start L16
  constraint midpoint L24.end L2
  constraint midpoint L11.start L10
  constraint midpoint L11.end L26
  constraint midpoint L13.start L22
  constraint midpoint L13.end L15
  constraint tangent L24 A0
  constraint tangent L11 A0
  measures "d330_1" distance of L3 L19
extrude "cap body'" add sketch "Road Cap Curve" along normal blind 4.8 separate body contours L0 L2 L7 L8 L10 L16 L20 L23 L25 L26 A1 | L10 L20 A1 A3 | L2 L8 A1 A3 | L10 L20 A0 A3 | L7 L8 L20 L23 L25 A1 | L8 L20 A1 A3 | L2 L8 A0 A3 | L10 L20 A0 A4 | L8 L20 A0 A3 | L2 L8 A0 A4 | L10 L20 A2 A4 | L8 L20 A0 A4 | L2 L8 A2 A4 | L2 L4 L8 L10 L20 L21 A2 | L8 L20 A2 A4 | L4 L8 L20 A2 | L1 L5 L14 L15 L17 L22 | L3 L6 L9 L12 L18 L19 makes body 6 in component "Road Cap Curve"
extrude "top lip cut'" cut sketch "Road Cap Curve" against normal blind 1.8 from surface at 4.8 contours L1 L5 L14 L15 L17 L22 | L3 L6 L9 L12 L18 L19 bodies 6 in component "Road Cap Curve"
extrude "Interior Hole" cut sketch "Road Cap Curve" along normal blind 2 contours L0 L2 L7 L8 L10 L16 L20 L23 L25 L26 A1 | L10 L20 A1 A3 | L2 L8 A1 A3 | L10 L20 A0 A3 | L7 L8 L20 L23 L25 A1 | L8 L20 A1 A3 | L2 L8 A0 A3 | L10 L20 A0 A4 | L8 L20 A0 A3 | L2 L8 A0 A4 | L10 L20 A2 A4 | L8 L20 A0 A4 | L2 L8 A2 A4 | L2 L4 L8 L10 L20 L21 A2 | L8 L20 A2 A4 | L4 L8 L20 A2 | L1 L5 L14 L15 L17 L22 bodies 6 in component "Road Cap Curve"
sketch "Road Cap Bridge" plane through (0, 0, 0) normal (0, 0, 1) x (1, 0, 0) in component "Road Cap Bridge"
  line L0 (106.7167, 11.795) -> (99.7885, -0.205)
  line L1 (120.6309, 11.895) -> (106.659, 11.895)
  line L2 (106.7167, -12.205) -> (120.5731, -12.205)
  line L3 (104.1706, -16.615) -> (123.1192, -16.615)
  line L4 (120.0535, -11.305) -> (126.4621, -0.205)
  line L5 (99.6731, -0.205) -> (106.659, -12.305)
  line L6 (94.6963, -0.205) -> (104.1706, -16.615)
  line L7 (100.8278, -0.205) -> (107.2363, -11.305)
  line L8 (107.2363, -11.305) -> (120.0535, -11.305)
  line L9 (132.5936, -0.205) -> (123.1192, 16.205)
  line L10 (127.5013, -0.205) -> (120.5731, 11.795)
  line L11 (124.0372, 5.795) -> (103.2526, -6.205) construction
  line L12 (104.1706, 16.205) -> (94.6963, -0.205)
  line L13 (103.166, 5.845) -> (124.1238, -6.255) construction
  line L14 (106.659, -12.305) -> (120.6309, -12.305)
  line L15 (120.6309, -12.305) -> (127.6168, -0.205)
  line L16 (120.5731, 11.795) -> (106.7167, 11.795)
  line L17 (127.6168, -0.205) -> (120.6309, 11.895)
  line L18 (123.1192, -16.615) -> (132.5936, -0.205)
  line L19 (123.1192, 16.205) -> (104.1706, 16.205)
  line L20 (126.4621, -0.205) -> (120.0535, 10.895)
  line L21 (120.5731, -12.205) -> (127.5013, -0.205)
  line L22 (106.659, 11.895) -> (99.6731, -0.205)
  line L23 (120.0535, 10.895) -> (107.2363, 10.895)
  line L24 (113.6449, 11.795) -> (113.6449, -12.205) construction
  line L25 (107.2363, 10.895) -> (100.8278, -0.205)
  line L26 (99.7885, -0.205) -> (106.7167, -12.205)
  line L27 (101.532, -1.4249) -> (120.7578, 9.6751)
  line L28 (125.7578, 1.0149) -> (106.532, -10.0851)
  line L29 (107.2363, 10.895) -> (120.0535, -11.305) construction
  line L30 (101.732, -1.7713) -> (120.9578, 9.3287)
  line L31 (101.332, -1.0785) -> (120.5578, 10.0215)
  line L32 (125.5578, 1.3613) -> (106.332, -9.7387)
  line L33 (125.9578, 0.6685) -> (106.732, -10.4315)
  line L34 (109.652, 6.7273) -> (108.1449, 4.1333)
  line L35 (108.1449, 4.1333) -> (109.6379, 1.5311)
  line L36 (109.6379, 1.5311) -> (112.6379, 1.523)
  line L37 (112.6379, 1.523) -> (114.1449, 4.117)
  line L38 (114.1449, 4.117) -> (112.652, 6.7191)
  line L39 (112.652, 6.7191) -> (109.652, 6.7273)
  line L40 (117.6517, -7.1293) -> (119.1449, -4.5273)
  line L41 (119.1449, -4.5273) -> (117.6381, -1.9331)
  line L42 (117.6381, -1.9331) -> (114.6381, -1.941)
  line L43 (114.6381, -1.941) -> (113.1449, -4.543)
  line L44 (113.1449, -4.543) -> (114.6517, -7.1371)
  line L45 (114.6517, -7.1371) -> (117.6517, -7.1293)
  point P0 (113.6449, -0.205)
  point P1 (110.0406, 6.0378)
  point P2 (111.1449, 4.1251)
  point P3 (116.1449, -4.5351)
  dimension "d328_2" = 0.1
  dimension "d330_2" = 32.82
  dimension "d377" = 10
  dimension "d378" = 0.4
  dimension "d380" = 0.4
  dimension "d383" = 3
  dimension "d384" = 3
  constraint horizontal L19
  constraint midpoint L24.start L16
  constraint midpoint L24.end L2
  constraint midpoint L11.start L10
  constraint midpoint L11.end L26
  constraint midpoint L13.start L22
  constraint midpoint L13.end L15
  constraint coincident L7 L27.start
  constraint coincident L20 L27.end
  constraint perpendicular L20 L27
  constraint coincident L20 L28.start
  constraint coincident L7 L28.end
  constraint perpendicular L7 L28
  constraint symmetric L11 L27 L28
  constraint midpoint L27 P2
  constraint midpoint L28 P3
  measures "d330_2" distance of L3 L19
  measures "d377" distance of L27 L28
  measures "d383" distance of L34.start P2
  measures "d384" distance of L40.start P3
extrude "cap body''" add sketch "Road Cap Bridge" along normal blind 4.8 separate body contours L0 L2 L10 L16 L21 L26 | L1 L5 L14 L15 L17 L22 | L3 L6 L9 L12 L18 L19 | L4 L7 L8 L20 L33 L40 L41 L44 L45 | L20 L28 L33 L41 | L7 L28 L33 L44 | L20 L28 L32 L41 | L33 L40 L41 L44 L45 | L28 L33 L41 L44 | L7 L28 L32 L44 | L7 L20 L30 L32 L35 L36 L37 L38 L41 L42 L43 L44 | L28 L32 L41 L44 | L20 L27 L30 L38 | L32 L41 L42 L43 L44 | L7 L27 L30 L35 | L20 L27 L31 L38 | L30 L35 L36 L37 L38 | L27 L30 L35 L38 | L7 L27 L31 L35 | L7 L20 L23 L25 L31 L34 L35 L38 L39 | L27 L31 L35 L38 | L31 L34 L35 L38 L39 makes body 7 in component "Road Cap Bridge"
extrude "top lip cut''" cut sketch "Road Cap Bridge" against normal blind 1.8 from surface at 4.8 contours L1 L5 L14 L15 L17 L22 | L3 L6 L9 L12 L18 L19 bodies 7 in component "Road Cap Bridge"
extrude "road cut" cut sketch "Road Cap" against normal blind 1.2 from surface at 4.8 contours L4 L7 L8 L20 L28 | L7 L20 L23 L25 L27 bodies 5 in component "Road Cap"
extrude "Extrude7" cut sketch "Road Cap" against normal blind 0.4 from surface at 4.8 contours L7 L20 L29 L30 bodies 5 in component "Road Cap"
extrude "Extrude8'" cut sketch "Road Cap" along normal blind 1.8 contours L0 L2 L10 L16 L21 L26 | L1 L5 L14 L15 L17 L22 | L4 L7 L8 L20 L28 | L7 L20 L28 L30 | L7 L20 L29 L30 | L7 L20 L27 L29 | L7 L20 L23 L25 L27 bodies 5 in component "Road Cap"
extrude "Internal hole cut" cut sketch "Road Cap Bridge" along normal blind 1.8 contours L0 L2 L10 L16 L21 L26 | L1 L5 L14 L15 L17 L22 | L4 L7 L8 L20 L33 L40 L41 L44 L45 | L20 L28 L33 L41 | L7 L28 L33 L44 | L20 L28 L32 L41 | L33 L40 L41 L44 L45 | L28 L33 L41 L44 | L7 L28 L32 L44 | L7 L20 L30 L32 L35 L36 L37 L38 L41 L42 L43 L44 | L28 L32 L41 L44 | L20 L27 L30 L38 | L32 L41 L42 L43 L44 | L7 L27 L30 L35 | L20 L27 L31 L38 | L30 L35 L36 L37 L38 | L27 L30 L35 L38 | L7 L27 L31 L35 | L7 L20 L23 L25 L31 L34 L35 L38 L39 | L27 L31 L35 L38 | L31 L34 L35 L38 L39 bodies 7 in component "Road Cap Bridge"
extrude "road cut'" cut sketch "Road Cap Bridge" against normal blind 1.2 from surface at 4.8 contours L4 L7 L8 L20 L33 L40 L41 L44 L45 | L7 L20 L23 L25 L31 L34 L35 L38 L39 bodies 7 in component "Road Cap Bridge"
extrude "Extrude9'" cut sketch "Road Cap Bridge" against normal blind 0.4 from surface at 4.8 contours L7 L20 L30 L32 L35 L36 L37 L38 L41 L42 L43 L44 | L32 L41 L42 L43 L44 | L30 L35 L36 L37 L38 bodies 7 in component "Road Cap Bridge"
extrude "road cut''" cut sketch "Road Cap Curve" against normal blind 1.2 from surface at 4.8 contours L7 L8 L20 L23 L25 A1 | L4 L8 L20 A2 bodies 6 in component "Road Cap Curve"
extrude "Extrude8''" cut sketch "Road Cap Curve" against normal blind 0.4 from surface at 4.8 contours L8 L20 A0 A3 | L8 L20 A0 A4 bodies 6 in component "Road Cap Curve"
sketch "Road Junction Right" plane through (0, 0, 0) normal (0, 0, 1) x (1, 0, 0) in component "Road Juntcion right"
  line L0 (106.7167, 11.7437) -> (99.7885, -0.2563)
  line L1 (120.6309, 11.8437) -> (106.659, 11.8437)
  line L2 (106.7167, -12.2563) -> (120.5731, -12.2563)
  line L3 (104.1706, -16.6663) -> (123.1192, -16.6663)
  line L4 (120.0535, -11.3563) -> (126.4621, -0.2563)
  line L5 (99.6731, -0.2563) -> (106.659, -12.3563)
  line L6 (94.6963, -0.2563) -> (104.1706, -16.6663)
  line L7 (100.8278, -0.2563) -> (107.2363, -11.3563)
  line L8 (107.2363, -11.3563) -> (120.0535, -11.3563)
  line L9 (132.5936, -0.2563) -> (123.1192, 16.1537)
  line L10 (127.5013, -0.2563) -> (120.5731, 11.7437)
  line L11 (124.0372, 5.7437) -> (103.2526, -6.2563) construction
  line L12 (104.1706, 16.1537) -> (94.6963, -0.2563)
  line L13 (103.166, 5.7937) -> (124.1238, -6.3063) construction
  line L14 (106.659, -12.3563) -> (120.6309, -12.3563)
  line L15 (120.6309, -12.3563) -> (127.6168, -0.2563)
  line L16 (120.5731, 11.7437) -> (106.7167, 11.7437)
  line L17 (127.6168, -0.2563) -> (120.6309, 11.8437)
  line L18 (123.1192, -16.6663) -> (132.5936, -0.2563)
  line L19 (123.1192, 16.1537) -> (104.1706, 16.1537)
  line L20 (126.4621, -0.2563) -> (120.0535, 10.8437)
  line L21 (120.5731, -12.2563) -> (127.5013, -0.2563)
  line L22 (106.659, 11.8437) -> (99.6731, -0.2563)
  line L23 (120.0535, 10.8437) -> (107.2363, 10.8437)
  line L24 (113.6449, 11.7437) -> (113.6449, -12.2563) construction
  line L25 (107.2363, 10.8437) -> (100.8278, -0.2563)
  line L26 (99.7885, -0.2563) -> (106.7167, -12.2563)
  line L27 (101.532, -1.4762) -> (120.7578, 9.6238)
  line L28 (106.532, -10.1364) -> (125.7578, 0.9636)
  line L29 (101.732, -1.8226) -> (120.9578, 9.2774)
  line L30 (106.332, -9.79) -> (125.5578, 1.31)
  line L31 (125.7578, -1.4762) -> (106.532, 9.6238)
  line L32 (120.7578, -10.1364) -> (101.532, 0.9636)
  line L33 (125.5578, -1.8226) -> (106.332, 9.2774)
  line L34 (120.9578, -9.79) -> (101.732, 1.31)
  point P0 (113.6449, -0.2563)
  dimension "d328_3" = 0.1
  dimension "d330_3" = 32.82
  dimension "d366_1" = 10
  dimension "d369_1" = 0.4
  dimension "d405" = 10
  dimension "d407" = 0.4
  constraint horizontal L19
  constraint midpoint L24.start L16
  constraint midpoint L24.end L2
  constraint midpoint L11.start L10
  constraint midpoint L11.end L26
  constraint midpoint L13.start L22
  constraint midpoint L13.end L15
  constraint coincident L7 L27.start
  constraint coincident L20 L27.end
  constraint perpendicular L20 L27
  constraint coincident L7 L28.start
  constraint coincident L20 L28.end
  constraint perpendicular L20 L28
  constraint symmetric L11 L27 L28
  constraint coincident L4 L31.start
  constraint coincident L25 L31.end
  constraint perpendicular L25 L31
  constraint coincident L4 L32.start
  constraint coincident L25 L32.end
  constraint perpendicular L25 L32
  constraint symmetric L13 L31 L32
  measures "d330_3" distance of L3 L19
  measures "d366_1" distance of L27 L28
  measures "d405" distance of L31 L32
extrude "Cap body" add sketch "Road Junction Right" along normal blind 4.8 separate body contours L0 L2 L10 L16 L21 L26 | L1 L5 L14 L15 L17 L22 | L3 L6 L9 L12 L18 L19 | L4 L7 L8 L28 L32 | L4 L28 L32 L34 | L4 L28 L33 L34 | L28 L30 L32 L34 | L7 L28 L30 L32 | L4 L28 L31 L33 | L28 L30 L33 L34 | L29 L30 L32 L34 | L7 L29 L30 L32 | L4 L20 L28 L31 | L28 L30 L31 L33 | L29 L30 L33 L34 | L27 L29 L32 L34 | L7 L27 L29 L32 | L20 L28 L30 L31 | L29 L30 L31 L33 | L27 L29 L33 L34 | L25 L27 L32 L34 | L7 L25 L27 L32 | L20 L29 L30 L31 | L27 L29 L31 L33 | L25 L27 L33 L34 | L20 L27 L29 L31 | L25 L27 L31 L33 | L20 L23 L25 L27 L31 makes body 8 in component "Road Juntcion right"
extrude "top lip cut'''" cut sketch "Road Junction Right" against normal blind 1.8 from surface at 4.8 contours L1 L5 L14 L15 L17 L22 | L3 L6 L9 L12 L18 L19 bodies 8 in component "Road Juntcion right"
extrude "Cap internal hole" cut sketch "Road Junction Right" along normal blind 2 contours L0 L2 L10 L16 L21 L26 | L1 L5 L14 L15 L17 L22 | L4 L7 L8 L28 L32 | L4 L28 L32 L34 | L4 L28 L33 L34 | L28 L30 L32 L34 | L7 L28 L30 L32 | L4 L28 L31 L33 | L28 L30 L33 L34 | L29 L30 L32 L34 | L7 L29 L30 L32 | L4 L20 L28 L31 | L28 L30 L31 L33 | L29 L30 L33 L34 | L27 L29 L32 L34 | L7 L27 L29 L32 | L20 L28 L30 L31 | L29 L30 L31 L33 | L27 L29 L33 L34 | L25 L27 L32 L34 | L7 L25 L27 L32 | L20 L29 L30 L31 | L27 L29 L31 L33 | L25 L27 L33 L34 | L20 L27 L29 L31 | L25 L27 L31 L33 | L20 L23 L25 L27 L31 bodies 8 in component "Road Juntcion right"
extrude "Road Cut" cut sketch "Road Junction Right" against normal blind 1.2 from surface at 4.8 contours L4 L7 L8 L28 L32 | L4 L20 L28 L31 | L25 L27 L32 L34 | L7 L25 L27 L32 | L25 L27 L33 L34 | L25 L27 L31 L33 | L20 L23 L25 L27 L31 bodies 8 in component "Road Juntcion right"
extrude "Road Indent" cut sketch "Road Junction Right" against normal blind 0.4 from surface at 4.8 contours L4 L28 L33 L34 | L28 L30 L33 L34 | L29 L30 L32 L34 | L7 L29 L30 L32 | L29 L30 L33 L34 | L29 L30 L31 L33 | L20 L29 L30 L31 bodies 8 in component "Road Juntcion right"